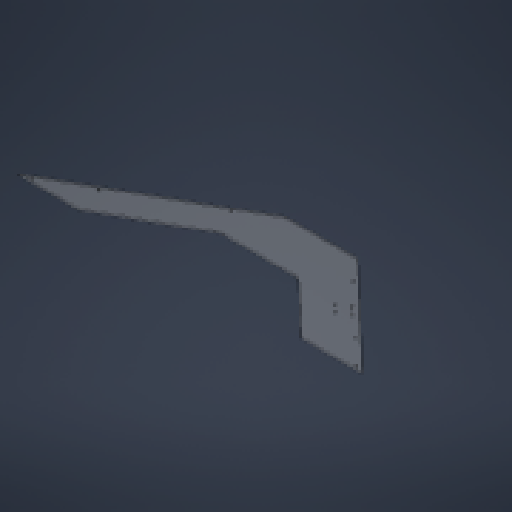
# Autodesk Inventor part: hopper_back
Saved by Autodesk Inventor 2024.3 (Build 283343000, 343)
## iProperties
Created: 2025-03-07
Part Number: hopper_back
Material: Polycarbonate, Clear
Document SubType Name: Sheet Metal
Designer: marcu
Density: 1.2 g/cm^3
Sheet Metal Rule: Default
Appearance: Polycarbonate - Clear
Mass: 418.486 g
Surface Area: 2356.23 cm^2
Volume: 348.738 cm^3
Author: marcu
Autodesk Inventor part; units mm, degrees
ref_plane "YZ Plane" through (0, 0, 0) normal (1, 0, 0) x (0, 1, 0)
ref_plane "XZ Plane" through (0, 0, 0) normal (0, 1, 0) x (-1, 0, 0)
ref_plane "XY Plane" through (0, 0, 0) normal (0, 0, 1) x (1, 0, 0)
ref_plane "Work Plane1" through (-1041.8338, 286.0261, 217.3698) normal (0, 0.9659258, -0.258819) x (0.7071068, -0.1830127, -0.6830127)
sketch "Sketch1" plane through (-1041.8338, 286.0261, 217.3698) normal (0, 0.9659258, -0.258819) x (0.7071068, -0.1830127, -0.6830127)
  line L0 (110.8111, -517.2111) -> (110.8111, -110.8111) construction
  line L1 (109.9183, -108.6558) -> (2.1553, -0.8927) construction
  line L2 (107.7631, -517.2111) -> (-203.2, -206.248) construction
  line L3 (2.1553, -0.8927) -> (110.8111, -109.5486)
  line L4 (110.8111, -109.5486) -> (110.8111, -517.2111)
  line L5 (110.8111, -517.2111) -> (107.7631, -517.2111)
  line L6 (107.7631, -517.2111) -> (-203.2, -206.248)
  line L7 (56.4832, -55.2206) -> (-148.8721, -260.5759) construction
  line L8 (110.8111, -109.5486) -> (2.1553, -0.8927)
  line L9 (2.1553, -0.8927) -> (-405.5073, -0.8927)
  line L10 (-405.5073, -0.8927) -> (-405.5073, -3.9407)
  line L11 (-405.5073, -3.9407) -> (-94.5442, -314.9038)
  line L12 (110.8111, -109.5486) -> (155.7124, -64.6473)
  line L13 (155.7124, -64.6473) -> (47.0565, 44.0085)
  line L14 (47.0565, 44.0085) -> (2.1553, -0.8927)
  line L15 (2.1553, -0.8927) -> (110.8111, -109.5486)
  line L16 (-41.109, -368.339) -> (-41.109, -169.5133)
  line L17 (-57.8095, -152.8128) -> (-256.6352, -152.8128)
  arc A0 (-41.109, -169.5133) -> (-57.8095, -152.8128) centre (-57.8095, -169.5133) ccw
  line L18 (151.2222, -60.1571) -> (110.8111, -100.5683)
  line L19 (110.8111, -100.5683) -> (110.8111, -109.5486)
  line L20 (51.5467, 39.5184) -> (11.1355, -0.8927)
  line L21 (11.1355, -0.8927) -> (2.1553, -0.8927)
  point P0 (937.5005, -535.875)
  point P1 (2.1553, -0.8927)
  point P2 (-203.2, -206.248)
  point P3 (110.8111, -109.5486)
  point P4 (-256.6352, -152.8128)
  point P5 (-41.109, -368.339)
  point P6 (-41.109, -152.8128)
  point P7 (110.8111, -109.5486)
  point P8 (2.1553, -0.8927)
  point P9 (110.8111, -109.5486)
  dimension "d1" = 63.5
  dimension "d62" = 152.4
  dimension "d63" = 16.7005
  dimension "d65" = 6.35
  measures "d1" distance of L8.start L12.end
  measures "d62" distance from line of L2 point (-41.109, -152.813)
  measures "d63" radius of A0
  measures "d65" distance between parallel lines of L18 L12
extrude "Plate1" add sketch "Sketch1" along normal blind 3.048 contours L21 L20 L13 L18 L19 L3 | L3 L4 L5 L6 L16 A0 L17 L11 L10 L9
sketch "Sketch2" plane through (-1041.8338, 288.9702, 216.5809) normal (0, 0.9659258, -0.258819) x (0.7071068, 0.1830127, 0.6830127)
  line L0 (-39.5184, 51.5467) -> (60.1571, 151.2222) construction
  line L1 (60.1571, 151.2222) -> (94.8324, 116.5469) construction
  line L2 (10.3194, 101.3844) -> (24.957, 86.7468) construction
  line L3 (60.1571, 151.2222) -> (100.5683, 110.8111) projected
  point P0 (535.875, 937.5005)
  point P1 (42.8728, 104.752)
  point P2 (6.9518, 68.831)
  point P3 (-44.0085, 47.0565)
  point P4 (56.3432, 91.2817)
  point P5 (20.4222, 55.3606)
  dimension "d2" = 20.6375
  dimension "d3" = 20.6375
  dimension "d4" = 50.8
  dimension "d7" = 19.05
  dimension "d12" = 25.4
  constraints: 4 end point, 1 collinear, 1 midpoint, 1 perpendicular, 3 other
  measures "d2" distance from line of point (42.873, 104.752) L0
  measures "d3" distance from line of L0 point (6.952, 68.831)
  measures "d4" distance of point (6.952, 68.831) point (42.873, 104.752)
  measures "d7" distance of point (42.873, 104.752) point (56.343, 91.282)
  measures "d12" distance from line of L2 point (42.873, 104.752)
hole "Hole1" at (-937.4473, 277.6455, 174.3166) at (-988.2473, 277.6455, 174.3166) at (-937.4473, 282.576, 192.7175) at (-988.2473, 282.576, 192.7175) direction (0, -0.9659258, 0.258819) diameter 5.1054 end through all clearance for "Flat Head Machine Screw (82)" size "#10" standard "Ansi Unified Screw Threads"
sketch "Sketch3" plane through (-1041.8338, 288.9702, 216.5809) normal (0, 0.9659258, -0.258819) x (0.7071068, 0.1830127, 0.6830127)
  line L0 (517.2111, 110.8111) -> (517.2111, 107.7631) construction
  line L1 (100.5683, 110.8111) -> (517.2111, 110.8111) construction
  line L2 (0.8927, -405.5073) -> (0.8927, 11.1355) construction
  line L3 (3.9407, -405.5073) -> (0.8927, -405.5073) construction
  line L4 (517.2111, 107.7631) -> (368.339, -41.109) construction
  line L5 (192.5185, 283.5836) -> (442.775, 33.327) construction
  line L6 (308.8897, 110.8111) -> (308.8897, 98.1111) construction
  line L7 (109.5486, 110.8111) -> (517.2111, 110.8111) construction
  line L8 (152.8128, -256.6352) -> (3.9407, -405.5073) projected
  line L9 (152.8128, -57.8095) -> (152.8128, -256.6352) projected
  line L10 (368.339, -41.109) -> (169.5133, -41.109) projected
  line L11 (-39.5184, 51.5467) -> (60.1571, 151.2222) projected
  arc A0 (169.5133, -41.109) -> (152.8128, -57.8095) centre (169.5133, -57.8095) ccw projected
  line L12 (60.1571, 151.2222) -> (100.5683, 110.8111) projected
  line L13 (0.8927, 11.1355) -> (-39.5184, 51.5467) projected
  point P0 (535.875, 937.5005)
  point P1 (283.4897, 98.1111)
  point P2 (308.8897, 72.7111)
  point P3 (283.4897, 72.7111)
  point P4 (377.991, 167.2124)
  point P5 (377.991, 192.6124)
  point P6 (403.391, 167.2124)
  point P7 (403.391, 192.6124)
  dimension "d20" = 12.7
  dimension "d23" = 25.4
  dimension "d26" = 25.4
  constraints: 4 end point, 4 symmetric about line, 2 midpoint, 2 perpendicular, 1 coincident, 1 horizontal, 1 vertical, 3 other
  measures "d20" distance of L6.start L6.end
  measures "d23" distance of point (308.89, 98.111) point (283.49, 98.111)
  measures "d26" distance of point (308.89, 98.111) point (308.89, 72.711)
hole "Hole2" at (-754.0408, 327.5454, 360.5454) at (-772.0013, 322.8969, 343.1969) at (-772.0013, 332.1939, 377.8939) at (-789.9618, 327.5454, 360.5454) at (-638.3563, 332.1939, 377.8939) at (-620.3958, 327.5454, 360.5454) at (-656.3168, 327.5454, 360.5454) at (-638.3563, 322.8969, 343.1969) direction (0, -0.9659258, 0.258819) diameter 5.1054 end through all clearance for "Flat Head Machine Screw (82)" size "#10" standard "Ansi Unified Screw Threads"
ref_plane "Work Plane2" through (-962.8473, 265.9096, 142.2942) normal (1, 0, 0) x (0, -0.9659258, 0.258819)
sketch "Sketch5" plane through (-1041.8338, 288.9702, 216.5809) normal (0, 0.9659258, -0.258819) x (0.7071068, 0.1830127, 0.6830127)
  line L0 (100.5683, 110.8111) -> (517.2111, 110.8111) projected
  line L1 (517.2111, 101.9084) -> (109.471, 101.9084) construction
  line L2 (517.2111, 110.8111) -> (517.2111, 107.7631) projected
  line L3 (60.1571, 151.2222) -> (100.5683, 110.8111) projected
  point P0 (535.875, 937.5005)
  point P1 (498.1611, 101.9084)
  point P2 (396.5611, 101.9084)
  point P3 (193.3611, 101.9084)
  point P4 (109.5486, 110.8111)
  dimension "d40" = 8.9027
  dimension "d41" = 101.6
  dimension "d42" = 19.05
  dimension "d45" = 203.2
  constraints: 5 point on line, 2 end point, 1 parallel
  measures "d40" distance between parallel lines of L0 L1
  measures "d41" distance of point (498.161, 101.908) point (396.561, 101.908)
  measures "d42" distance of L1.start point (498.161, 101.908)
  measures "d45" distance of point (396.561, 101.908) point (193.361, 101.908)
hole "Hole3" at (-617.5206, 361.4895, 487.2266) at (-689.3626, 342.8954, 417.8325) at (-833.0467, 305.7072, 279.0443) direction (0, -0.9659258, 0.258819) diameter 5.1054 end through all
mirror "Mirror2" about plane through (-962.8473, 265.9096, 142.2942) normal (1, 0, 0) of "Hole3", "Hole2"
equation "\"d3\" = d2"
equation "\"d18\" = Thickness"
equation "\"d51\" = Thickness"
equation "\"d0\" = Thickness"
equation "\"BendRadius\" = Thickness"
equation "\"BendReliefWidth\" = Thickness"
equation "\"BendReliefDepth\" = 0.5 * Thickness"
equation "\"CornerReliefSize\" = 4 * Thickness"
equation "\"MinimumRemnant\" = 2 * Thickness"
equation "\"TransitionRadius\" = BendRadius"
equation "\"JacobiRadiusSize\" = BendRadius"
equation "\"GapSize\" = Thickness"
equation "\"Thickness\" = 3.048"
body "Solid1"
